opener (Autodesk Fusion 360 design; units mm, degrees)
Autodesk Fusion 360 part; units mm, degrees
sketch "Sketch1" plane through (0, 0, 0) normal (0, 1, 0) x (1, 0, 0)
  line L0 (8.4913, -39.1738) -> (-41.5087, -39.1738)
  arc A0 (-78.8921, -12.4892) -> (-41.5087, -39.1738) centre (-41.5087, 0.3543) ccw
  spline S0 degree 5 poles (-78.8921, -12.4892) (-77.0371, -12.4344) (-73.42, -12.4447) (-68.2728, -12.8201) (-61.9809, -13.9861) (-55.1226, -16.2272) (-49.3004, -18.815) (-44.4641, -21.2819) (-40.4469, -23.2051) (-36.8893, -24.2963) (-33.2774, -24.4453) (-29.3096, -23.6289) (-25.2026, -21.8441) (-22.0239, -19.0326) (-20.99, -15.1728) (-22.8452, -10.36) (-27.0687, -4.911) (-32.1979, 0.691) (-36.406, 5.8907) (-38.0066, 10.1417) (-35.9554, 12.9896) (-30.4417, 14.1641) (-22.5735, 13.5769) (-13.9236, 11.304) (-6.1079, 7.5765) (-0.393, 2.7633) (2.8117, -2.6302) (4.0295, -8.0148) (4.276, -12.8308) (4.758, -16.6435) (6.5084, -19.2509) (10.0725, -20.7747) (15.6102, -21.5337) (22.9762, -21.9311) (31.8085, -22.3348) (41.6102, -22.9667) (51.7866, -23.9325) (61.684, -25.2441) (70.6275, -26.8453) (77.9585, -28.6349) (83.0738, -30.4917) (85.4619, -32.2975) (84.7456, -33.9632) (80.6653, -35.4263) (73.0554, -36.6455) (61.8244, -37.5969) (49.9114, -38.1346) (39.3263, -38.4106) (31.5367, -38.5382) (27.4587, -38.5878) knots 0 0 0 0 0 0 0.022222 0.044444 0.066667 0.088889 0.111111 0.133333 0.155556 0.177778 0.2 0.222222 0.244444 0.266667 0.288889 0.311111 0.333333 0.355556 0.377778 0.4 0.422222 0.444444 0.466667 0.488889 0.511111 0.533333 0.555556 0.577778 0.6 0.622222 0.644444 0.666667 0.688889 0.711111 0.733333 0.755556 0.777778 0.8 0.822222 0.844444 0.866667 0.888889 0.911111 0.933333 0.955556 0.977778 1 1 1 1 1 1
  line L1 (-99.066, -13.0852) -> (-58.7182, -11.8932)
  line L2 (27.4587, -38.5878) -> (8.4913, -39.1738)
  point P0 (-41.6041, -22.5702)
  point P1 (-29.3309, -23.4023)
  point P2 (-21.8421, -14.0414)
  point P3 (-37.0276, 10.297)
  point P4 (-3.3283, 4.8885)
  point P5 (4.9925, -16.1216)
  point P6 (82.7921, -30.683)
  point P7 (22.9044, -21.9083)
  dimension "d1" = 50
  dimension "d2" = 109.5063
  constraint horizontal L0
  constraint tangent L0 A0
  constraint midpoint A0.start L1
  measures "d1" distance of L0.start L0.end
  measures "d2" distance of A0.start S0.end
extrude "Extrude1" add sketch "Sketch1" along normal blind 25
ref_plane "WorkPlane1" through (2.9821, 12.5, 12.6951) normal (0, -1, 0) x (-1, 0, 0)
sketch "Sketch2" plane through (2.9821, 12.5, 12.6951) normal (0, -1, 0) x (1, 0, 0)
  line L0 (-35, -10) -> (-17, -10)
  line L1 (-17, -10) -> (-17, -11.4)
  line L2 (-17, -11.4) -> (-35, -11.4)
  line L3 (-35, -11.4) -> (-35, -10)
  line L4 (-32, -10) -> (-32, -11.4)
  dimension "d5" = 18
  dimension "d6" = 1.4
  dimension "d7" = 3
  constraint horizontal L0
  constraint vertical L1
  constraint horizontal L2
  constraint vertical L3
  constraint coincident L0 L4.start
  constraint coincident L2 L4.end
  constraint perpendicular L2 L4
  measures "d5" distance of L0.start L0.end
  measures "d6" distance of L0.start L2.end
  measures "d7" distance of L3 L4
extrude "Extrude2" cut sketch "Sketch2" along normal mid plane 16
sketch "Sketch7" plane through (0, 0, 0) normal (0, 1, 0) x (1, 0, 0)
sketch "Sketch4" plane through (0, 0, 0) normal (0, 1, 0) x (1, 0, 0)
